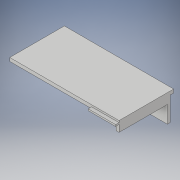
# Autodesk Inventor part: Wire Housing Wall vglue
Saved by Autodesk Inventor 2019 (Build 230136000, 136)
## iProperties
Created: 2020-03-06
Part Number: Wire Housing Wall vglue
Material: Generic
Document SubType Name: Modeling
Designer: Obscure_Decision
Density: 1 g/cm^3
Appearance: Default
Author: Obscure_Decision
Autodesk Inventor part; units mm, degrees
ref_plane "YZ Plane" through (0, 0, 0) normal (1, 0, 0) x (0, 1, 0)
ref_plane "XZ Plane" through (0, 0, 0) normal (0, 1, 0) x (-1, 0, 0)
ref_plane "XY Plane" through (0, 0, 0) normal (0, 0, 1) x (1, 0, 0)
sketch "Sketch1" plane through (0, 0, 0) normal (0, 1, 0) x (-1, 0, 0)
  line L0 (50.8, 25.4) -> (-50.8, 25.4)
  line L1 (-50.8, 25.4) -> (-50.8, -25.4)
  line L2 (-50.8, -25.4) -> (50.8, -25.4)
  line L3 (50.8, -25.4) -> (50.8, 25.4)
  line L4 (50.8, 25.4) -> (-50.8, -25.4) construction
  line L5 (-50.8, 25.4) -> (50.8, -25.4) construction
  point P0 (0, 0)
  dimension "d0" = 101.6
  dimension "d1" = 50.8
  constraints: 12 end point, 2 midpoint, 2 parallel, 1 horizontal, 1 perpendicular
  measures "d0" distance of L2.end L1.end
  measures "d1" distance of L1.end L0.end
extrude "Extrusion1" add sketch "Sketch1" along normal blind 3.175
sketch "Sketch3" plane through (0, 3.175, 0) normal (0, 1, 0) x (1, 0, 0)
  line L0 (50.8, 25.4) -> (-50.8, 25.4) projected
  line L1 (0, 25.4) -> (0, 22.098) construction
  line L2 (-50.8, 25.4) -> (-50.8, -25.4) construction
  line L3 (-50.8, 25.4) -> (-50.8, -25.4) construction
  line L4 (-50.8, 25.4) -> (-47.498, 25.4) construction
  line L5 (-47.498, 25.4) -> (-47.498, -25.4) construction
  line L6 (-50.8, -25.4) -> (50.8, -25.4) construction
  line L7 (-47.498, 22.098) -> (50.8, 22.098) construction
  line L8 (50.8, -25.4) -> (50.8, 25.4) projected
  line L9 (-47.498, 22.098) -> (50.8, 22.098)
  line L10 (50.8, 22.098) -> (50.8, 19.558)
  line L11 (50.8, 19.558) -> (-47.498, 19.558)
  line L12 (-47.498, 19.558) -> (-47.498, 22.098)
  point P0 (0, 0)
  dimension "d8" = 3.302
  dimension "d9" = 3.302
  dimension "d10" = 2.54
  constraints: 18 end point, 4 point on line, 2 horizontal, 2 parallel, 2 perpendicular, 2 vertical, 1 midpoint
  measures "d8" distance of L1.start L1.end
  measures "d9" distance of L0.end L4.end
  measures "d10" distance of L9.end L10.end
extrude "Extrusion3" add sketch "Sketch3" against normal blind 25.4
sketch "Sketch4" plane through (0, 3.175, 0) normal (0, 1, 0) x (1, 0, 0)
  line L0 (50.8, 19.558) -> (-47.498, 19.558) projected
  line L1 (-50.8, -25.4) -> (50.8, -25.4) projected
  line L2 (50.8, 19.558) -> (48.26, 19.558)
  line L3 (48.26, 19.558) -> (48.26, -25.4)
  line L4 (48.26, -25.4) -> (50.8, -25.4)
  line L5 (50.8, -25.4) -> (50.8, 19.558)
  point P0 (0, 0)
  dimension "d13" = 2.54
  constraints: 8 end point, 2 parallel, 1 horizontal, 1 perpendicular, 1 point on line
  measures "d13" distance of L4.end L3.end
extrude "Extrusion4" add sketch "Sketch4" against normal blind 9.525
sketch "Sketch5" plane through (-50.8, 3.175, 25.4) normal (0, 0, 1) x (1, 0, 0)
  line L0 (101.6, -3.175) -> (0, -3.175) projected
  line L1 (101.6, -3.175) -> (76.2, -3.175)
  line L2 (76.2, -3.175) -> (76.2, -1.651)
  line L3 (76.2, -1.651) -> (101.6, -1.651)
  line L4 (101.6, -1.651) -> (101.6, -3.175)
  point P0 (50.8, -3.175)
  dimension "d16" = 25.4
  dimension "d17" = 1.524
  constraints: 8 end point, 2 parallel, 1 horizontal, 1 perpendicular
  measures "d16" distance of L2.end L3.end
  measures "d17" distance of L1.end L2.end
extrude "Extrusion5" add sketch "Sketch5" along normal blind 3.175
body "Solid1"
